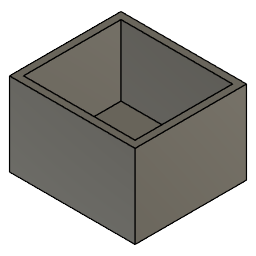
drawer (Autodesk Fusion 360 design; units mm, degrees)
part number: 2026-07-15-19-35-30-879
Autodesk Fusion 360 part; units mm, degrees
sketch "Sketch4" plane through (0, 0, 0) normal (0, 0, 1) x (1, 0, 0)
  line L0 (0, 30) -> (89.0049, 30)
  line L1 (89.0049, 30) -> (89.0049, -49)
  line L2 (89.0049, -49) -> (0, -49)
  line L3 (0, -49) -> (0, 30)
  dimension "d3" = 79
  constraint horizontal L0
  constraint vertical L1
  constraint horizontal L2
  constraint vertical L3
  measures "d3" distance of L0.start L2.end
sketch "Sketch5" plane through (0, 0, 0) normal (0, 0, 1) x (1, 0, 0)
  line L0 (5, 25) -> (84, 25)
  line L1 (84, 25) -> (84, -44)
  line L2 (84, -44) -> (5, -44)
  line L3 (5, -44) -> (5, 25)
  constraint horizontal L0
  constraint vertical L1
  constraint horizontal L2
  constraint vertical L3
extrude "Extrude1" add sketch "Sketch4" sketch "Sketch5" along normal blind 59 of sketch 2
extrude "Extrude2" cut sketch "Sketch5" along normal blind 50
move_body "Move1" bodies 1 to x (-1, 0, 0) y (0, 1, 0) z (0, 0, -1) at (109.0141, 0, 79.1446)
